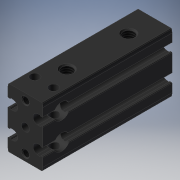
# Autodesk Inventor part: 4674228 DPDM-15---(h)
Saved by Autodesk Inventor 2019 (Build 230136000, 136)
## iProperties
Created: 2024-05-27
Part Number: 4674228 DPDM-15---(h)
Material: Generic
Catalog Web Link: www.cadenas.de
Description: DPDM(h)-housing
Vendor: FESTO
Document SubType Name: Modeling
Designer: psAdmin
Manufacturer: FESTO
Mass: 10.0128 g
Surface Area: 62.5754 cm^2
Volume: 10.0128 cm^3
Density: 1 g/cm^3
Appearance: PSOLRGB-175-175-175
Category: PARTsolutions
Company: FESTO
Title: 4674228 DPDM-15---(h)
Author: Cadenas PARTsolutions
Comments: housing
PSOL_IDENT_0: {$CADENAS_DATA/23d-libs/festo/parts/d/dpdm/parts/dpdm_housing.prj},201 {VTYP=3D},{NB=4674228 DPDM-15
PSOL_IDENT_1: ---(h)},{LINA=4674228 DPDM-15---(h)},{NN=DPDM(h)},{DATE=23.02.2024 06:49:52},{GEOMDATE=23.02.2024 06
PSOL_IDENT_2: :49:00},{VERSION=},{LINEID=10},{WBVAR=VER,HUB,FUN,KOT},{WBNUMERIC=HUB}  {NB=4674228 DPDM-15---(h)},{
PSOL_IDENT_3: LINA=4674228 DPDM-15---(h)},{KT=DUMMY},{TNR=4674228},{TYP=DPDM},{VER=-},{VERNB=},{KOL=6},{HUB=15},{H
PSOL_IDENT_4: UB1=5,10,15,20,25,30},{FUN=-},{FUN1='-','P','S'},{FUNNB=},{KOT=-},{KOT1='-','T'},{KOTNB=},{MM=3.000}
PSOL_IDENT_5: ,{L2=33.000},{EE=M5},{EEN=5.000},{ET=4.000},{BG=5.000},{RT=M3},{RTN=3.000},{H2=10.000},{E=13.000},{U
PSOL_IDENT_6: O=22.000},{TO=17.000},{H3=7.000},{LX=7.000},{PL=17.500},{PR=9.600},{U1=0.000},{D5=3.300},{D6=6.000},
PSOL_IDENT_7: {T1=5.000},{A1X=4.200},{A1Y=1.400},{A2X=2.810},{A2Y=4.710},{W2=3.000},{R1=0.000},{A3=0.000},{L1=19.3
PSOL_IDENT_8: 5},{L3=7.000},{DQ=3.000}
NB: 4674228 DPDM-15---(h)
NN: DPDM(h)
NT: housing
NBSYN: $TNR. $TYP.$VERNB.-$HUB.$FUNNB.$KOTNB.---(h)
LINA: 4674228 DPDM-15---(h)
CATALOG: Festo
TNR: 4674228
TYP: DPDM
VER: -
KOL: 6
HUB: 15
FUN: -
KOT: -
MM: 3
L2: 33
EE: M5
EEN: 5
ET: 4
BG: 5
RT: M3
RTN: 3
H2: 10
E: 13
UO: 22
TO: 17
H3: 7
LX: 7
PL: 17.5
PR: 9.6
U1: 0
D5: 3.3
D6: 6
T1: 5
A1X: 4.2
A1Y: 1.4
A2X: 2.81
A2Y: 4.71
W2: 3
R1: 0
A3: 0
L3: 7
DQ: 3
SUPPLIER: FESTO
ARTICLENO: 4674228 DPDM-15---(h)
BOMINFO: 4674228 DPDM-15---(h)
CREATOR: CADENAS GmbH
Autodesk Inventor part; units mm, degrees
sketch "Sketch_1" plane through (0, 0, 0) normal (0, 0, 1) x (1, 0, 0)
  line L0 (-6.5, -11) -> (6.5, -11)
  line L1 (6.5, -11) -> (6.5, 11)
  line L2 (6.5, 11) -> (-6.5, 11)
  line L3 (-6.5, 11) -> (-6.5, -11)
  constraints: 8 end point
extrude "Extrusion1" add sketch "Sketch_1" against normal blind 48
sketch "Sketch_2" plane through (0, 0, 0) normal (0, 0, 1) x (1, 0, 0)
  line L0 (-16.5, -21) -> (16.5, -21)
  line L1 (16.5, -21) -> (16.5, 21)
  line L2 (16.5, 21) -> (-16.5, 21)
  line L3 (-16.5, 21) -> (-16.5, -21)
  line L4 (-6.5, 3.1906) -> (-6.5, -3.1906)
  arc A0 (-6.5, -3.1906) -> (-6.2895, -3.3903) centre (-6.3, -3.1906) ccw
  line L5 (-6.2895, -3.3903) -> (-5.8644, -3.368)
  arc A1 (-5.8644, -3.368) -> (-5.6941, -3.1785) centre (-5.8738, -3.1883) ccw
  arc A2 (-5.4865, -2.9679) -> (-5.6941, -3.1785) centre (-5.4944, -3.1677) ccw
  line L6 (-5.4865, -2.9679) -> (-4.5361, -3.0056)
  arc A3 (-4.3484, -6.5855) -> (-4.5361, -3.0056) centre (-4.6075, -4.8042) ccw
  line L7 (-4.3484, -6.5855) -> (-5.2897, -6.7224)
  arc A4 (-5.5182, -6.5346) -> (-5.2897, -6.7224) centre (-5.3185, -6.5245) ccw
  arc A5 (-5.5182, -6.5346) -> (-5.7074, -6.3639) centre (-5.698, -6.5437) ccw
  line L8 (-5.7074, -6.3639) -> (-6.3105, -6.3955)
  arc A6 (-6.3105, -6.3955) -> (-6.5, -6.5952) centre (-6.3, -6.5952) ccw
  line L9 (-6.5, -6.5952) -> (-6.5, -9.6)
  arc A7 (-6.5, -9.6) -> (-6.3295, -10.7846) centre (-2.3, -9.6) ccw
  arc A8 (-6.3295, -10.7846) -> (-6.0417, -11) centre (-6.0417, -10.7) ccw
  line L10 (-6.0417, -11) -> (6.0417, -11)
  arc A9 (6.0417, -11) -> (6.3295, -10.7846) centre (6.0417, -10.7) ccw
  arc A10 (6.3295, -10.7846) -> (6.5, -9.6) centre (2.3, -9.6) ccw
  line L11 (6.5, -9.6) -> (6.5, -6.5952)
  arc A11 (6.5, -6.5952) -> (6.3105, -6.3955) centre (6.3, -6.5952) ccw
  line L12 (6.3105, -6.3955) -> (5.7074, -6.3639)
  arc A12 (5.7074, -6.3639) -> (5.5182, -6.5346) centre (5.698, -6.5437) ccw
  arc A13 (5.2897, -6.7224) -> (5.5182, -6.5346) centre (5.3185, -6.5245) ccw
  line L13 (5.2897, -6.7224) -> (4.3484, -6.5855)
  arc A14 (4.5361, -3.0056) -> (4.3484, -6.5855) centre (4.6075, -4.8042) ccw
  line L14 (4.5361, -3.0056) -> (5.4865, -2.9679)
  arc A15 (5.6941, -3.1785) -> (5.4865, -2.9679) centre (5.4944, -3.1677) ccw
  arc A16 (5.6941, -3.1785) -> (5.8644, -3.368) centre (5.8738, -3.1883) ccw
  line L15 (5.8644, -3.368) -> (6.2895, -3.3903)
  arc A17 (6.2895, -3.3903) -> (6.5, -3.1906) centre (6.3, -3.1906) ccw
  line L16 (6.5, -3.1906) -> (6.5, 3.1906)
  arc A18 (6.5, 3.1906) -> (6.2895, 3.3903) centre (6.3, 3.1906) ccw
  line L17 (6.2895, 3.3903) -> (5.8644, 3.368)
  arc A19 (5.8644, 3.368) -> (5.6941, 3.1785) centre (5.8738, 3.1883) ccw
  arc A20 (5.4865, 2.9679) -> (5.6941, 3.1785) centre (5.4944, 3.1677) ccw
  line L18 (5.4865, 2.9679) -> (4.5361, 3.0056)
  arc A21 (4.3484, 6.5855) -> (4.5361, 3.0056) centre (4.6075, 4.8042) ccw
  line L19 (4.3484, 6.5855) -> (5.2897, 6.7224)
  arc A22 (5.5182, 6.5346) -> (5.2897, 6.7224) centre (5.3185, 6.5245) ccw
  arc A23 (5.5182, 6.5346) -> (5.7074, 6.3639) centre (5.698, 6.5437) ccw
  line L20 (5.7074, 6.3639) -> (6.3105, 6.3955)
  arc A24 (6.3105, 6.3955) -> (6.5, 6.5952) centre (6.3, 6.5952) ccw
  line L21 (6.5, 6.5952) -> (6.5, 9.6)
  arc A25 (6.5, 9.6) -> (6.3295, 10.7846) centre (2.3, 9.6) ccw
  arc A26 (6.3295, 10.7846) -> (6.0417, 11) centre (6.0417, 10.7) ccw
  line L22 (6.0417, 11) -> (-6.0417, 11)
  arc A27 (-6.0417, 11) -> (-6.3295, 10.7846) centre (-6.0417, 10.7) ccw
  arc A28 (-6.3295, 10.7846) -> (-6.5, 9.6) centre (-2.3, 9.6) ccw
  line L23 (-6.5, 9.6) -> (-6.5, 6.5952)
  arc A29 (-6.5, 6.5952) -> (-6.3105, 6.3955) centre (-6.3, 6.5952) ccw
  line L24 (-6.3105, 6.3955) -> (-5.7074, 6.3639)
  arc A30 (-5.7074, 6.3639) -> (-5.5182, 6.5346) centre (-5.698, 6.5437) ccw
  arc A31 (-5.2897, 6.7224) -> (-5.5182, 6.5346) centre (-5.3185, 6.5245) ccw
  line L25 (-5.2897, 6.7224) -> (-4.3484, 6.5855)
  arc A32 (-4.5361, 3.0056) -> (-4.3484, 6.5855) centre (-4.6075, 4.8042) ccw
  line L26 (-4.5361, 3.0056) -> (-5.4865, 2.9679)
  arc A33 (-5.6941, 3.1785) -> (-5.4865, 2.9679) centre (-5.4944, 3.1677) ccw
  arc A34 (-5.6941, 3.1785) -> (-5.8644, 3.368) centre (-5.8738, 3.1883) ccw
  line L27 (-5.8644, 3.368) -> (-6.2895, 3.3903)
  arc A35 (-6.2895, 3.3903) -> (-6.5, 3.1906) centre (-6.3, 3.1906) ccw
  constraints: 72 point on circle, 56 end point, 36 centre point
extrude "Extrusion2" cut sketch "Sketch_2" against normal blind 48
sketch "Sketch_6" plane through (0, 0, 0) normal (1, 0, 0) x (0, 1, 0)
  line L0 (0, -33.65) -> (0, 0)
  line L1 (0, 0) -> (1.5, 0)
  line L2 (1.5, 0) -> (1.5, -13.65)
  line L3 (1.5, -13.65) -> (3, -13.65)
  line L4 (3, -13.65) -> (3, -33.65)
  line L5 (3, -33.65) -> (0, -33.65)
  line L6 (0, -33.65) -> (0, 0)
  constraints: 14 end point
revolve "Revolution1" cut sketch "Sketch_6" angle 360 about axis through (0, 0, -33.65) along (0, 0, -1)
sketch "Sketch4" plane through (0, 0, -48) normal (0, 0, -1) x (-1, 0, 0)
  point P0 (0, 0)
hole "Hole1" at (0, 0, -48) direction (0, 0, 1) diameter 7 depth 0.5 countersink diameter 7.4 countersink angle 90
sketch "Sketch_9" plane through (0, 0, 0) normal (1, 0, 0) x (0, 1, 0)
  line L0 (3.7783, -15.5) -> (11, -15.5)
  line L1 (11, -15.5) -> (11, -18)
  line L2 (11, -18) -> (10.567, -17.567)
  line L3 (10.567, -17.567) -> (6, -17.567)
  line L4 (6, -17.567) -> (6, -16.75)
  line L5 (6, -16.75) -> (4.5, -16.75)
  line L6 (4.5, -16.75) -> (3.7783, -15.5)
  line L7 (3.7783, -15.5) -> (11, -15.5)
  constraints: 16 end point
revolve "Revolution2" cut sketch "Sketch_9" angle 360 about axis through (0, 3.7783, -15.5) along (0, -1, 0)
thread "Thread1" size "M5x0.8" class "6H" standard "ISO Metric profile" length 3.567
pattern_linear "Rectangular Pattern1" count 2 spacing 22.9 along (0, 0, -1) of "Revolution2"
sketch "Sketch6" plane through (0, 0, -48) normal (0, 0, -1) x (-1, 0, 0)
  point P0 (0, 8.5)
hole "Hole2" at (0, 8.5, -48) direction (0, 0, 1) diameter 2.459 depth 6 countersink diameter 3 countersink angle 90 thread size "M3x0.5" class "6H" standard "ISO Metric profile"
pattern_linear "Rectangular Pattern2" count 2 spacing 17 along (0, -1, 0) of "Hole2"
sketch "Sketch7" plane through (0, 0, 0) normal (0, 0, 1) x (1, 0, 0)
  point P0 (0, 8.5)
hole "Hole3" at (0, 8.5, 0) direction (0, 0, -1) diameter 2.459 depth 6 countersink diameter 3 countersink angle 90 thread size "M3x0.5" class "6H" standard "ISO Metric profile"
sketch "Sketch8" plane through (0, 0, 0) normal (0, 0, 1) x (1, 0, 0)
  point P0 (0, -8.5)
hole "Hole4" at (0, -8.5, 0) direction (0, 0, -1) diameter 2.459 depth 6 countersink diameter 3 countersink angle 90 thread size "M3x0.5" class "6H" standard "ISO Metric profile"
sketch "Sketch9" plane through (-6.0417, -11, 0) normal (0, -1, 0) x (1, 0, 0)
  point P0 (9.5417, -7)
hole "Hole5" at (3.5, -11, -7) direction (0, 1, 0) diameter 3.3 depth 22
pattern_linear "Rectangular Pattern3" count 2 spacing 7 along (-1, 0, 0) of "Hole5"
sketch "Sketch_28" plane through (0, 0, -7) normal (0, 0, 1) x (1, 0, 0)
  line L0 (6.5, 5) -> (-6.5, 5)
  line L1 (-6.5, 5) -> (-6.5, 8)
  line L2 (-6.5, 8) -> (-1.5, 8)
  line L3 (-1.5, 8) -> (-1.5, 6.65)
  line L4 (-1.5, 6.65) -> (1.5, 6.65)
  line L5 (1.5, 6.65) -> (1.5, 8)
  line L6 (1.5, 8) -> (6.5, 8)
  line L7 (6.5, 8) -> (6.5, 5)
  line L8 (6.5, 5) -> (-6.5, 5)
  constraints: 18 end point
revolve "Revolution3" cut sketch "Sketch_28" angle 360 about axis through (6.5, 5, -7) along (1, 0, 0)
pattern_linear "Rectangular Pattern4" count 2 spacing 10 along (0, -1, 0) of "Revolution3"
ref_plane "ANBAU_XY" through (0, 0, 0) normal (0, 0, 1) x (1, 0, 0)
ref_plane "ANBAU_YZ" through (0, 0, 0) normal (1, 0, 0) x (0, 1, 0)
ref_plane "ANBAU_ZX" through (0, 0, 0) normal (0, 1, 0) x (0, 0, 1)
ref_plane "CP_DR_XY" through (0, 11, -38.4) normal (0, -1, 0) x (1, 0, 0)
ref_plane "CP_DR_YZ" through (0, 11, -38.4) normal (1, 0, 0) x (0, 0, 1)
ref_plane "CP_DR_ZX" through (0, 11, -38.4) normal (0, 0, 1) x (0, -1, 0)
ref_plane "CP_ROD1_XY" through (0, 0, -33.65) normal (0, 0, 1) x (1, 0, 0)
ref_plane "CP_ROD1_YZ" through (0, 0, -33.65) normal (1, 0, 0) x (0, 1, 0)
ref_plane "CP_ROD1_ZX" through (0, 0, -33.65) normal (0, 1, 0) x (0, 0, 1)
ref_plane "CP_ROD_P_XY" through (0, 0, -33.65) normal (0, 0, -1) x (1, 0, 0)
ref_plane "CP_ROD_P_YZ" through (0, 0, -33.65) normal (1, 0, 0) x (0, -1, 0)
ref_plane "CP_ROD_P_ZX" through (0, 0, -33.65) normal (0, -1, 0) x (0, 0, -1)
ref_plane "SCHRAUBE_1_XY" through (1.5, 5, -7) normal (-1, 0, 0) x (0, 0, -1)
ref_plane "SCHRAUBE_1_YZ" through (1.5, 5, -7) normal (0, 0, -1) x (0, -1, 0)
ref_plane "SCHRAUBE_1_ZX" through (1.5, 5, -7) normal (0, -1, 0) x (-1, 0, 0)
ref_plane "SCHRAUBE_2_XY" through (1.5, -5, -7) normal (-1, 0, 0) x (0, 0, -1)
ref_plane "SCHRAUBE_2_YZ" through (1.5, -5, -7) normal (0, 0, -1) x (0, -1, 0)
ref_plane "SCHRAUBE_2_ZX" through (1.5, -5, -7) normal (0, -1, 0) x (-1, 0, 0)
ref_plane "SCHRAUBE_B_1_XY" through (3.5, 11, -7) normal (0, -1, 0) x (1, 0, 0)
ref_plane "SCHRAUBE_B_1_YZ" through (3.5, 11, -7) normal (1, 0, 0) x (0, 0, 1)
ref_plane "SCHRAUBE_B_1_ZX" through (3.5, 11, -7) normal (0, 0, 1) x (0, -1, 0)
ref_plane "SCHRAUBE_B_2_XY" through (-3.5, 11, -7) normal (0, -1, 0) x (1, 0, 0)
ref_plane "SCHRAUBE_B_2_YZ" through (-3.5, 11, -7) normal (1, 0, 0) x (0, 0, 1)
ref_plane "SCHRAUBE_B_2_ZX" through (-3.5, 11, -7) normal (0, 0, 1) x (0, -1, 0)
ref_plane "TO_QSML_1_XY" through (0, 11, -15.5) normal (0, -1, 0) x (0, 0, -1)
ref_plane "TO_QSML_1_YZ" through (0, 11, -15.5) normal (0, 0, -1) x (1, 0, 0)
ref_plane "TO_QSML_1_ZX" through (0, 11, -15.5) normal (1, 0, 0) x (0, -1, 0)
ref_plane "TO_QSML_2_XY" through (0, 11, -38.4) normal (0, -1, 0) x (0, 0, -1)
ref_plane "TO_QSML_2_YZ" through (0, 11, -38.4) normal (0, 0, -1) x (1, 0, 0)
ref_plane "TO_QSML_2_ZX" through (0, 11, -38.4) normal (1, 0, 0) x (0, -1, 0)
body "Solid1"
